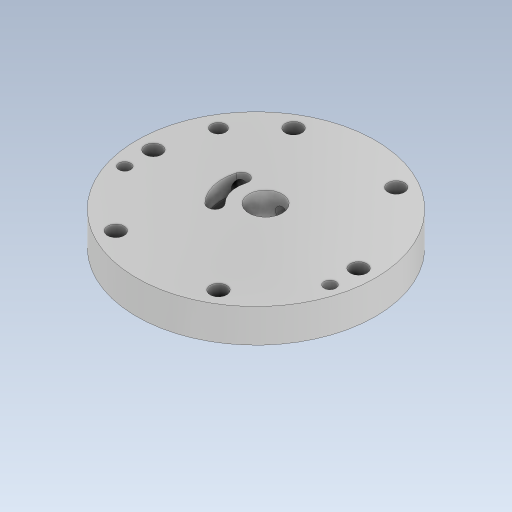
# Autodesk Inventor part: Pump-Motor-CW-Rotation:Casing 102
Saved by Autodesk Inventor 2024.2 (Build 282272000, 272)
## iProperties
Created: 2025-06-16
Material: Aluminum 6061
Document SubType Name: Modeling
Density: 2.7 g/cm^3
Appearance: Aluminum - Polished
Designer: cw
Author: cw
Autodesk Inventor part; units mm, degrees
note: some values were not read from the file. Chosen so that the rebuilt part matches the saved one: direction of "Hole5".
ref_plane "YZ Plane" through (0, 0, 0) normal (1, 0, 0) x (0, 1, 0)
sketch "Sketch1" plane through (0, 0, 0) normal (0, 0, 1) x (1, 0, 0)
  circle A0 centre (0, 0) radius 50
  dimension "d0" = 100
  constraints: 1 centre point, 1 coincident
  measures "d0" diameter of A0
extrude "Extrusion1" add sketch "Sketch1" along normal blind 14
sketch "Sketch2" plane through (0, 0, 0) normal (0, 0, -1) x (-1, 0, 0)
  circle A0 centre (0, 4) radius 23
  point P0 (0, 0)
  dimension "d3" = 46
  dimension "d4" = 4
  constraints: 1 centre point, 1 vertical alignment
  measures "d3" diameter of A0
  measures "d4" distance of A0.centre point (0, 0)
extrude "Extrusion2" add sketch "Sketch2" along normal blind 20
sketch "Sketch3" plane through (0, 4, -20) normal (0, 0, -1) x (-1, 0, 0)
  circle A0 centre (0, 0) radius 23 construction
  point P0 (0, -4)
hole "Hole1" at (0, 4, -20) direction (0, 0, 1) diameter 14 end through all counterbore diameter 28 counterbore depth 21
sketch "Sketch4" plane through (0, 4, -20) normal (0, 0, -1) x (-1, 0, 0)
  circle A0 centre (0, 0) radius 14 projected
  point P0 (0, -4)
hole "Hole2" at (0, 4, -20) direction (0, 0, 1) diameter 33.835 depth 13 thread size "M36x2" class "6H" standard "ISO Metric profile"
sketch "Sketch5" plane through (0, 0, 14) normal (0, 0, 1) x (1, 0, 0)
  circle A0 centre (0, 0) radius 43 construction
  point P0 (-43, 0)
  dimension "d21" = 86
  constraints: 2 horizontal alignment, 1 coincident, 2 other
hole "Hole3" at (-43, 0, 14) direction (0, 0, -1) diameter 7 end through all
pattern_circular "Circular Pattern1" count 6 over 360 about axis through (0, 0, 0) along (0, 0, 1) of "Hole3"
sketch "Sketch6" plane through (0, 0, 14) normal (0, 0, 1) x (1, 0, 0)
  circle A0 centre (-43, 0) radius 3.5 construction
  circle A1 centre (43, 0) radius 3.5 construction
  point P0 (0, 0)
  point P1 (-43, -12)
  point P2 (43, -12)
  dimension "d32" = 12
  constraints: 2 vertical alignment, 1 horizontal alignment
  measures "d32" distance of A1.centre point (43, -12)
hole "Hole4" at (-43, -12, 14) at (43, -12, 14) direction (0, 0, -1) diameter 5 depth 6 tip angle 118
sketch "Sketch7" plane through (0, 0, 14) normal (0, 0, 1) x (1, 0, 0)
  circle A0 centre (0, 0) radius 43 construction
  line L0 (0, 0) -> (-37.2391, 21.5) construction
  line L1 (-70, 0) -> (70, 0) construction
  circle A1 centre (-37.2391, 21.5) radius 3
  circle A2 centre (0, 4) radius 7 construction
  arc A3 (-14.3713, 8.2973) -> (-10.6066, -6.6066) centre (0, 4) ccw construction
  arc A4 (-17.2455, 9.1567) -> (-12.7279, -8.7279) centre (0, 4) ccw
  arc A5 (-11.497, 7.4378) -> (-8.4853, -4.4853) centre (0, 4) ccw
  arc A6 (-11.497, 7.4378) -> (-17.2455, 9.1567) centre (-14.3713, 8.2973) ccw
  arc A7 (-12.7279, -8.7279) -> (-8.4853, -4.4853) centre (-10.6066, -6.6066) ccw
  line L2 (0, 4) -> (-10.6066, -6.6066) construction
  line L3 (0, 4) -> (-15, 4) construction
  dimension "d40" = 86
  dimension "d41" = 30
  dimension "d42" = 6
  dimension "d43" = 15
  dimension "d44" = 6
  dimension "d45" = 45
  constraints: 11 point on circle, 6 centre point, 6 end point, 4 tangent, 3 coincident, 1 horizontal, 1 point on line, 3 other
  measures "d41" angle of L1 L0
  measures "d42" diameter of A1
  measures "d43" radius of A3
  measures "d44" radial gap between concentric circles of A5 A4
  measures "d45" angle of L2 L3
extrude "Extrusion3" cut sketch "Sketch7" against normal blind 7.5
ref_plane "Work Plane1" through (0, 0, 9) normal (0, 0, 1) x (1, 0, 0)
sketch "Sketch8" plane through (0, 0, 9) normal (0, 0, 1) x (1, 0, 0)
  circle A0 centre (-37.2391, 21.5) radius 3 construction
  arc A1 (-11.497, 7.4378) -> (-17.2455, 9.1567) centre (-14.3713, 8.2973) ccw construction
  line L0 (-37.2391, 21.5) -> (-14.3713, 8.2973)
  line L1 (-14.3713, 8.2973) -> (-13.1213, 10.4623)
  line L2 (-13.1213, 10.4623) -> (-35.9891, 23.6651)
  line L3 (-35.9891, 23.6651) -> (-37.2391, 21.5)
  point P0 (0, 0)
  dimension "d49" = 5
  constraints: 8 end point, 2 parallel, 1 perpendicular
  measures "d49" diameter of L2 L0
revolve "Revolution1" cut sketch "Sketch8" angle 360 about axis through (-37.2391, 21.5, 9) along (0.8660254, -0.5, 0)
ref_plane "Work Plane2" through (0, 50, 0) normal (0, 1, 0) x (-1, 0, 0)
sketch "Sketch9" plane through (0, 50, 0) normal (0, 1, 0) x (-1, 0, 0)
  line L0 (50, 14) -> (-50, 14) construction
  point P0 (0, 0)
  point P1 (0, 7)
  dimension "d51" = 7
  constraints: 1 vertical alignment
  measures "d51" distance from line of point (0, 7) L0
hole "Hole5" at (0, 50, 7) direction (0, -1, 0) diameter 4.917 end up to surface counterbore diameter 13.5 counterbore depth 1 thread size "M6x1" class "6H" standard "ISO Metric profile"
sketch "Sketch10" plane through (0, 4, 1) normal (0, 0, -1) x (-1, 0, 0)
  circle A0 centre (0, 0) radius 7 projected
  circle A1 centre (0, 0) radius 12
  point P0 (0, -4)
  dimension "d59" = 24
  constraints: 1 centre point, 1 coincident
  measures "d59" diameter of A1
extrude "Extrusion4" cut sketch "Sketch10" against normal blind 1
body "Solid1"
